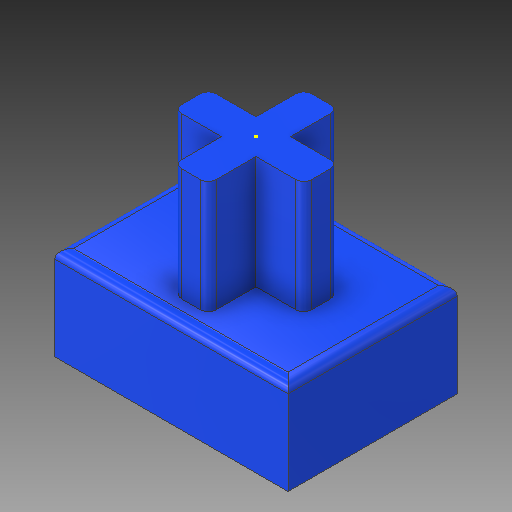
# Autodesk Inventor part: keyswitch-pole_cherrymx
Saved by Autodesk Inventor 2018 (Build 220112000, 112)
## iProperties
Created: 2016-12-08
Part Number: keyswitch-pole_cherrymx
Material: Generic
Document SubType Name: Modeling
Designer: Cemra JC
Density: 1 g/cm^3
Appearance: Default
Author: Cemra JC
Autodesk Inventor part; units mm, degrees
ref_plane "YZ Plane" through (0, 0, 0) normal (1, 0, 0) x (0, 1, 0)
ref_plane "XZ Plane" through (0, 0, 0) normal (0, 1, 0) x (-1, 0, 0)
ref_plane "XY Plane" through (0, 0, 0) normal (0, 0, 1) x (1, 0, 0)
sketch "Pole Base Profile" plane through (0, 0, 0) normal (0, 1, 0) x (-1, 0, 0)
  line L0 (3.725, 2.7) -> (-3.725, 2.7)
  line L1 (-3.725, 2.7) -> (-3.725, -2.7)
  line L2 (-3.725, -2.7) -> (3.725, -2.7)
  line L3 (3.725, -2.7) -> (3.725, 2.7)
  line L4 (3.725, 2.7) -> (-3.725, -2.7) construction
  line L5 (-3.725, 2.7) -> (3.725, -2.7) construction
  point P0 (0, 0)
  dimension "d0" = 7.45
  dimension "d1" = 5.4
  constraints: 12 end point, 2 midpoint, 2 parallel, 1 horizontal, 1 perpendicular
  measures "d0" distance of L1.end L2.end
  measures "d1" distance of L2.end L0.start
extrude "Pole Base" add sketch "Pole Base Profile" along normal blind 3
sketch "Cross Base" plane through (0, 3, 0) normal (0, 1, 0) x (1, 0, 0)
  line L0 (-0.55, -2.075) -> (0.55, -2.075)
  line L1 (0.55, -2.075) -> (0.55, 2.075)
  line L2 (0.55, 2.075) -> (-0.55, 2.075)
  line L3 (-0.55, 2.075) -> (-0.55, -2.075)
  line L4 (-0.55, -2.075) -> (0.55, 2.075) construction
  line L5 (0.55, -2.075) -> (-0.55, 2.075) construction
  line L6 (-2.075, -0.55) -> (2.075, -0.55)
  line L7 (2.075, -0.55) -> (2.075, 0.55)
  line L8 (2.075, 0.55) -> (-2.075, 0.55)
  line L9 (-2.075, 0.55) -> (-2.075, -0.55)
  line L10 (-2.075, -0.55) -> (2.075, 0.55) construction
  line L11 (2.075, -0.55) -> (-2.075, 0.55) construction
  point P0 (0, 0)
  dimension "d12" = 1.1
  dimension "d13" = 4.15
  dimension "d14" = 4.15
  dimension "d15" = 1.1
  constraints: 24 end point, 4 midpoint, 4 parallel, 2 horizontal, 2 perpendicular
  measures "d12" distance of L2.end L1.end
  measures "d13" distance of L1.end L0.end
  measures "d14" distance of L7.end L8.end
  measures "d15" distance of L6.end L7.end
extrude "Pole" add sketch "Cross Base" along normal blind 3.6
fillet "Pole Rounding" radius 0.25 8 edges at (2.075, 4.8, 0.55) (0.55, 4.8, 2.075) (-0.55, 4.8, 2.075) (-2.075, 4.8, 0.55) (-2.075, 4.8, -0.55) (-0.55, 4.8, -2.075) (0.55, 4.8, -2.075) (2.075, 4.8, -0.55)
fillet "Base Rounding" radius 0.3 4 edges at (-3.725, 3, 0) (0, 3, -2.7) (0, 3, 2.7) (3.725, 3, 0)
sketch "Top Center Point" plane through (0, 6.6, 0) normal (0, 1, 0) x (1, 0, 0)
  point P0 (0, 0)
equation "\"d0\" = s_polebl"
equation "\"d1\" = s_polebw"
equation "\"d12\" = k_cmxw"
equation "\"d13\" = k_cmxl"
equation "\"d14\" = d13"
equation "\"d15\" = d12"
equation "\"d8\" = s_poleh"
equation "\"k_width\" = 18"
equation "\"k_height\" = 16.5"
equation "\"k_taper1\" = 1.5"
equation "\"k_taper2\" = 0.5"
equation "\"k_radius\" = 6"
equation "\"k_wthick\" = 1.5"
equation "\"k_ribthick\" = 1.5"
equation "\"k_ribheight\" = 5"
equation "\"k_poleoff\" = 2.25"
equation "\"k_poledia\" = 5.3"
equation "\"k_cmxw\" = 1.1"
equation "\"k_cmxl\" = 4.15"
equation "\"s_bwidth\" = 14.4"
equation "\"s_poleh\" = 3.6"
equation "\"s_polebw\" = 5.4"
equation "\"s_polebl\" = 7.45"
equation "\"b_rshift\" = 49.5"
equation "\"b_height\" = 77"
equation "\"b_tab\" = 27"
equation "\"b_lshift\" = 40.5"
equation "\"b_space\" = 117"
equation "\"b_caps\" = 31.5"
equation "\"b_pad\" = 1"
equation "\"b_width\" = 285"
equation "\"b_ctrl\" = 22.5"
equation "\"k_staper\" = 1"
equation "\"k_ltaper\" = 1.5"
equation "\"k_sradius\" = 4"
equation "\"k_lradius\" = 6"
equation "\"k_height_t\" = 16"
equation "\"k_height_low\" = 15"
equation "\"k_taper_wide\" = 1.5"
equation "\"k_taper_thin\" = 0.0001"
equation "\"k_shortening\" = 4.5"
equation "\"k_cmxd\" = 4"
equation "\"k_taper_side\" = 0.5"
body "Solid1"
